Autodesk Fusion 360 part; units mm, degrees
(part 2 of 2)
  spline S354 degree 2 poles (-33.7284, -64.8766) (-33.9484, -65.013) (-34.0473, -65.2756) knots 0 0 0 1 1 1
  spline S355 degree 2 poles (-34.0473, -65.2756) (-34.1462, -65.5382) (-34.1462, -66.0328) knots 0 0 0 1 1 1
  line L236 (-34.1462, -66.0328) -> (-34.1462, -67.912)
  line L237 (-34.1462, -67.912) -> (-34.7601, -67.912)
  point P0 (0, -1)
  point P1 (0, -26)
  point P2 (0, -27)
  point P3 (-7.7833, -35.912)
  point P4 (8.2942, -35.912)
  point P5 (-7.7833, -40.7608)
  point P6 (8.2942, -40.7608)
  point P7 (-24.7058, -9.912)
  point P8 (-24.7058, -14.7608)
  point P9 (-40.7833, -14.7608)
  point P10 (-24.7058, -14.7608)
  point P11 (-40.7833, -9.912)
  point P12 (-40.7833, -14.7608)
  point P13 (-24.7058, -9.912)
  point P14 (-33, 0)
  point P15 (-40.7833, -9.912)
  point P16 (-33, -1)
  point P17 (-24.7058, -35.912)
  point P18 (-40.7833, -35.912)
  point P19 (-40.7833, -40.7608)
  point P20 (-40.7833, -40.7608)
  point P21 (-40.7833, -35.912)
  point P22 (-40.7833, -40.7608)
  point P23 (-40.7833, -35.912)
  point P24 (-24.7058, -40.7608)
  point P25 (-24.7058, -35.912)
  point P26 (-24.7058, -35.912)
  point P27 (-24.7058, -40.7608)
  point P28 (-33, -26)
  point P29 (-24.7058, -40.7608)
  point P30 (-33, -27)
  point P31 (32, 0)
  point P32 (32, -1)
  point P33 (24.2167, -9.912)
  point P34 (40.2942, -9.912)
  point P35 (24.2167, -14.7608)
  point P36 (40.2942, -14.7608)
  point P37 (40.2942, -35.912)
  point P38 (24.2167, -40.7608)
  point P39 (24.2167, -35.912)
  point P40 (32, -27)
  point P41 (32, -26)
  point P42 (40.2942, -40.7608)
  point P43 (24.2167, -35.912)
  point P44 (24.2167, -40.7608)
  point P45 (40.2942, -40.7608)
  point P46 (40.2942, -35.912)
  point P47 (-24.7058, -67.7608)
  point P48 (-40.7833, -67.7608)
  point P49 (-40.7833, -62.912)
  point P50 (-24.7058, -62.912)
  point P51 (-40.7833, -67.7608)
  point P52 (-40.7833, -62.912)
  point P53 (-24.7058, -62.912)
  point P54 (-40.7833, -62.912)
  point P55 (-24.7058, -62.912)
  point P56 (-24.7058, -67.7608)
  point P57 (-40.7833, -67.7608)
  point P58 (-33, -53)
  point P59 (-24.7058, -67.7608)
  point P60 (-24.7058, -67.7608)
  point P61 (-40.7833, -62.912)
  point P62 (-40.7833, -67.7608)
  point P63 (-24.7058, -62.912)
  point P64 (-33, -54)
  dimension "d1" = 30
  dimension "d3" = 12
  dimension "d4" = 12
  dimension "d5" = 3.5
  dimension "d18" = 30
  dimension "d19" = 12
  dimension "d20" = 12
  dimension "d21" = 3.5
  dimension "d23" = 30
  dimension "d24" = 12
  dimension "d25" = 12
  dimension "d26" = 3.5
  dimension "d28" = 30
  dimension "d29" = 12
  dimension "d30" = 12
  dimension "d31" = 3.5
  dimension "d33" = 30
  dimension "d34" = 12
  dimension "d35" = 12
  dimension "d36" = 3.5
  dimension "d38" = 30
  dimension "d39" = 12
  dimension "d40" = 12
  dimension "d41" = 3.5
  dimension "d43" = 30
  dimension "d44" = 12
  dimension "d45" = 12
  dimension "d46" = 3.5
  constraint parallel L0 L2
  constraint coincident L3 P0
  constraint coincident L4 P0
  constraint horizontal L6
  constraint perpendicular L6 L7
  constraint horizontal L8
  constraint perpendicular L8 L9
  constraint parallel L8 L10
  constraint parallel L9 L11
  constraint coincident L12 origin
  constraint coincident L13 origin
  constraint perpendicular L5 L14
  constraint parallel L18 L23
  constraint coincident P2 L20
  constraint coincident P2 L22
  constraint horizontal L28
  constraint perpendicular L27 L28
  constraint horizontal L24
  constraint perpendicular L16 L24
  constraint parallel L15 L24
  constraint parallel L16 L19
  constraint coincident P1 L26
  constraint coincident P1 L21
  constraint perpendicular L17 L25
  constraint parallel L41 L44
  constraint coincident P16 L36
  constraint coincident P16 L34
  constraint horizontal L40
  constraint perpendicular L37 L40
  constraint horizontal L39
  constraint perpendicular L38 L39
  constraint parallel L39 L42
  constraint parallel L32 L38
  constraint coincident P14 L33
  constraint coincident P14 L35
  constraint perpendicular L30 L31
  constraint parallel L46 L56
  constraint coincident P30 L45
  constraint coincident P30 L59
  constraint horizontal L57
  constraint perpendicular L49 L57
  constraint horizontal L55
  constraint perpendicular L52 L55
  constraint parallel L54 L55
  constraint parallel L48 L52
  constraint coincident P28 L50
  constraint coincident P28 L53
  constraint perpendicular L47 L58
  constraint parallel L68 L72
  constraint coincident P32 L69
  constraint coincident P32 L67
  constraint horizontal L73
  constraint perpendicular L71 L73
  constraint horizontal L63
  constraint perpendicular L63 L74
  constraint parallel L63 L64
  constraint parallel L60 L74
  constraint coincident P31 L62
  constraint coincident P31 L61
  constraint perpendicular L65 L70
  constraint parallel L87 L88
  constraint coincident P40 L76
  constraint coincident P40 L75
  constraint horizontal L78
  constraint perpendicular L78 L79
  constraint horizontal L86
  constraint perpendicular L84 L86
  constraint parallel L83 L86
  constraint parallel L81 L84
  constraint coincident P41 L82
  constraint coincident P41 L85
  constraint perpendicular L77 L89
  constraint parallel L93 L100
  constraint coincident P64 L95
  constraint coincident P64 L92
  constraint horizontal L97
  constraint perpendicular L97 L101
  constraint horizontal L99
  constraint perpendicular L96 L99
  constraint parallel L99 L104
  constraint parallel L96 L102
  constraint coincident P58 L91
  constraint coincident P58 L103
  constraint perpendicular L90 L94
  measures "d1" distance of L0.end L1.end
  measures "d3" distance of L9.end L10.end
  measures "d4" distance of L8.end L9.end
  measures "d5" diameter of A0
  measures "d18" distance of L18.start L20.end
  measures "d19" distance of L15.end L15.start
  measures "d20" distance of L15.start L16.start
  measures "d21" diameter of A2
  measures "d23" distance of L36.end L34.end
  measures "d24" distance of L33.end L32.start
  measures "d25" distance of L33.end L35.start
  measures "d26" diameter of A5
  measures "d28" distance of L45.end L51.end
  measures "d29" distance of L50.end L48.start
  measures "d30" distance of L50.end L52.start
  measures "d31" diameter of A6
  measures "d33" distance of L66.end L66.start
  measures "d34" distance of L60.start L62.end
  measures "d35" distance of L62.end L61.start
  measures "d36" diameter of A8
  measures "d38" distance of L75.end L76.end
  measures "d39" distance of L81.start L82.end
  measures "d40" distance of L84.start L82.end
  measures "d41" diameter of A11
  measures "d43" distance of L92.end L93.end
  measures "d44" distance of L102.start L91.end
  measures "d45" distance of L96.start L91.end
  measures "d46" diameter of A13
extrude "Extrude3" add sketch "Sketch1" along normal blind 1.8 contours L0 L1 L2 L5 L6 L7 L14 | L17 L18 L23 L25 L27 L28 L29 | L30 L31 L37 L40 L41 L43 L44 | L46 L47 L49 L51 L56 L57 L58 | L65 L66 L68 L70 L71 L72 L73 | L77 L78 L79 L80 L87 L88 L89 | L90 L93 L94 L97 L98 L100 L101 makes body 1 at (11.3526, -35.9848, 0) makes body 2 at (-43.8009, 5.2354, 0) makes body 3 at (-21.8032, -35.9848, 0) makes body 4 at (43.1968, -35.9848, 0) makes body 5 at (11.1968, -9.9848, 0) makes body 6 at (43.1968, -9.9848, 0) makes body 7 at (-22.0257, -61.0817, 0)
fillet "Fillet4" radius 3 8 edges at (-48, -42.5, 0.9) (-48, -18, 0.9) (-18, -18, 0.9) (-18, -42.5, 0.9) (-48, -69.5, 0.9) (-48, -45, 0.9) (-18, -45, 0.9) (-18, -69.5, 0.9) on bodies 3 7
fillet "Fillet5" radius 3 8 edges at (-48, 8, 0.9) (-48, -16.5, 0.9) (-18, 8, 0.9) (-18, -16.5, 0.9) (-15, 8, 0.9) (15, 8, 0.9) (-15, -16.5, 0.9) (15, -16.5, 0.9) on bodies 2 5
fillet "Fillet6" radius 3 12 edges at (-15, -18, 0.9) (15, -18, 0.9) (-15, -42.5, 0.9) (15, -42.5, 0.9) (17, -18, 0.9) (47, -18, 0.9) (47, -42.5, 0.9) (17, -42.5, 0.9) (17, 8, 0.9) (47, 8, 0.9) (17, -16.5, 0.9) (47, -16.5, 0.9) on bodies 1 4 6
